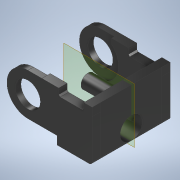
# Autodesk Inventor part: X-linear bearing shroud left half
Saved by Autodesk Inventor 2020 (Build 240168000, 168)
## iProperties
Created: 2021-02-25
Part Number: X-linear bearing shroud left half
Material: ABS Plastic
Document SubType Name: Modeling
Designer: AOB
Mass: 4.07668 g
Surface Area: 35.6097 cm^2
Volume: 3.84593 cm^3
Density: 1.06 g/cm^3
Appearance: Glossy - Black
Author: AOB
Autodesk Inventor part; units mm, degrees
ref_plane "YZ Plane" through (0, 0, 0) normal (1, 0, 0) x (0, 1, 0)
ref_plane "XZ Plane" through (0, 0, 0) normal (0, 1, 0) x (-1, 0, 0)
ref_plane "XY Plane" through (0, 0, 0) normal (0, 0, 1) x (1, 0, 0)
sketch "Sketch1" plane through (0, 0, 0) normal (0, 0, 1) x (1, 0, 0)
  line L0 (20.0398, 6.9501) -> (20.0361, 5.4501)
  line L1 (19.5349, 4.9513) -> (11.5349, 4.9713)
  line L2 (11.0361, 5.4725) -> (11.0399, 6.9725)
  line L3 (23.034, -6.5436) -> (23.034, 4.6148)
  line L4 (23.034, -6.5436) -> (23.034, -9.4606)
  line L5 (23.0412, 7.5) -> (23.034, 4.6148)
  arc A0 (22.034, -10.4606) -> (23.034, -9.4606) centre (22.034, -9.4606) ccw
  line L6 (23.0412, 7.5) -> (20.0398, 7.5)
  line L7 (5.0224, 7.5) -> (11.0399, 7.5)
  line L8 (5.0224, 7.5) -> (5.7962, 7.5)
  line L9 (20.0398, 6.9501) -> (20.0398, 7.5)
  line L10 (11.0399, 7.5) -> (11.0399, 6.9725)
  line L11 (20.0361, 5.4501) -> (19.5349, 4.9513)
  line L12 (11.0361, 5.4725) -> (11.5349, 4.9713)
  arc A1 (0, 7.5) -> (0.0224, -7.5) centre (0, 0) ccw
  line L13 (5.0224, 7.5) -> (0, 7.5)
  line L14 (0.0224, -7.5) -> (10.5134, -7.5)
  line L15 (22.034, -10.4606) -> (10.5134, -10.4606)
  line L16 (10.5134, -10.4606) -> (10.5134, -7.5)
  point P0 (20.0349, 4.9501)
  point P1 (11.0349, 4.9725)
  point P2 (23.0487, 10.4994)
  dimension "d3" = 1
  dimension "d47" = 10.491
  constraints: 34 end point, 6 point on line, 4 point on circle, 3 horizontal, 2 centre point, 2 parallel, 2 tangent, 2 vertical, 1 coincident, 1 perpendicular
  measures "d3" radius of A0
  measures "d47" distance of L14.start L14.end
extrude "Extrusion1" add sketch "Sketch1" along normal blind 3
sketch "Sketch3" plane through (0, 0, 0) normal (0, 0, -1) x (-1, 0, 0)
  line L0 (-23.0412, 7.5) -> (-20.0398, 7.5) projected
  line L1 (-23.0412, 7.5) -> (-20.0398, 7.5)
  line L2 (-20.0398, 7.5) -> (-20.0398, -7.5)
  line L3 (-20.0398, -7.5) -> (-10.4968, -7.5)
  line L4 (-10.727, -10.4606) -> (-22.034, -10.4606)
  arc A0 (-23.034, -9.4606) -> (-22.034, -10.4606) centre (-22.034, -9.4606) ccw projected
  line L5 (-23.034, -9.4606) -> (-23.034, -9.4606)
  line L6 (-23.034, -9.4606) -> (-23.0412, 7.5)
  arc A1 (-23.034, -9.4606) -> (-22.034, -10.4606) centre (-22.034, -9.4606) ccw
  line L7 (-10.727, -10.4606) -> (-10.4968, -10.4606)
  line L8 (-10.4968, -7.5) -> (-10.4968, -7.5)
  line L9 (-10.4968, -7.5) -> (-10.4968, -10.4606)
  dimension "d18" = 1
  dimension "d44" = 9.543
  constraints: 18 end point, 4 tangent, 3 perpendicular, 2 point on circle, 1 centre point, 1 horizontal, 1 vertical
  measures "d18" radius of A1
  measures "d44" distance of L8.start L2.end
extrude "Extrusion3" add sketch "Sketch3" along normal blind 11
ref_plane "Work Plane1" through (0, 0, -11) normal (0, 0, -1) x (-1, 0, 0)
sketch "Sketch4" plane through (20.0398, 6.9501, 0) normal (-1, 0, 0) x (0, 0, 1)
  circle A0 centre (-11, -6) radius 2.5
  point P0 (0, -6.9501)
  dimension "d22" = 5
  constraints: 1 centre point
  measures "d22" diameter of A0
extrude "Extrusion4" add sketch "Sketch4" along normal blind 12.5
sketch "Sketch6" plane through (0, 0, 0) normal (0, 0, -1) x (-1, 0, 0)
  arc A0 (-5.0224, 5.57) -> (0, 7.5) centre (0, 0) ccw
  arc A1 (5.0224, 5.5902) -> (0, 7.5) centre (0, -0.0589) ccw
  line L0 (-5.0224, 5.57) -> (-5.0224, 7.5)
  line L1 (-5.0224, 7.5) -> (-5.0224, 5.57)
  line L2 (-5.0224, 7.5) -> (0, 7.5) projected
  line L3 (-5.0224, 7.5) -> (0, 7.5)
  circle A2 centre (0, -0.0589) radius 4.5
  point P0 (5.0224, 5.5902)
  dimension "d37" = 9
  constraints: 6 end point, 4 point on circle, 3 centre point, 2 coincident, 2 collinear, 1 tangent, 1 vertical
  measures "d37" diameter of A2
extrude "Extrusion8" cut sketch "Sketch6" along normal mid plane 2 contours L0 L2 A0 | A2
extrude "Extrusion9" cut sketch "Sketch6" against normal through all contours A2
mirror "Mirror4" about plane through (0, 0, -11) normal (0, 0, -1) of "Extrusion1", "Extrusion3", "Extrusion8", "Extrusion9"
sketch "Sketch7" plane through (23.034, -9.4606, 0) normal (0.9999999, -0.0004249, 0) x (0, 0, -1)
  line L0 (0, -1.0053) -> (22, -1.0053) projected
  circle A0 centre (11, 3.4947) radius 4
  point P0 (0, 9.4508)
  dimension "d49" = 8
  constraints: 1 centre point
  measures "d49" diameter of A0
extrude "Extrusion10" cut sketch "Sketch7" against normal up to surface (12.5372 mm away)
body "Solid1"
